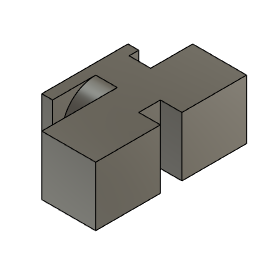
wire_screw v2 (Autodesk Fusion 360 design; units mm, degrees)
Autodesk Fusion 360 part; units mm, degrees
ref_plane "WorkPlane1" through (11.25, 0, 0) normal (1, 0, 0) x (0, 1, 0)
sketch "wire_screw2" plane through (0, 0, 0) normal (1, 0, 0) x (0, 1, 0)
  line L0 (7, 3.1) -> (-7, -3.1) construction
  line L1 (-7, 3.1) -> (7, -3.1) construction
  line L2 (-4, 4) -> (-4, -3.4897)
  line L3 (4, 4) -> (4, -3.5621)
  circle A0 centre (0, 0) radius 3.1
  circle A1 centre (0, 0) radius 2.75
  line L4 (-3.0288, -3.6864) -> (-3.0994, -0.0604)
  arc A2 (0, 2.75) -> (-3.0994, -0.0604) centre (0, -0.3643) ccw
  arc A3 (0, -2.75) -> (0, 2.75) centre (0, 0) ccw
  arc A4 (0, -2.75) -> (3.1, 0) centre (0, 0.3723) ccw
  line L5 (3.1, 0) -> (3.1, 3.8294)
  line L6 (0, 2.75) -> (3.1, 2.75)
  line L7 (0, -2.75) -> (-3.047, -2.75)
  line L8 (0, 2.75) -> (7, 2.75)
  line L9 (7, 2.75) -> (-7, 2.75)
  line L10 (-7, 2.75) -> (-7, -2.75)
  line L11 (-7, -2.75) -> (7, -2.75)
  line L12 (7, -2.75) -> (7, 2.75)
  dimension "d38" = 14
  dimension "d39" = 6.2
  dimension "d40" = 5.5
  dimension "d41" = 7
  dimension "d42" = 14
  constraint coincident A0.centre A1.centre
  constraint coincident L0 A0.centre
  constraint coincident L1 A0.centre
  constraint concentric A0 A1
  constraint coincident A0 L4.end
  constraint tangent A0 L4
  constraint tangent A1 A2
  constraint coincident A1 A2.start
  constraint tangent A1 A4
  constraint coincident A0 A4.end
  constraint tangent A0 L5
  constraint coincident L5 L6.end
  constraint tangent A1 L6
  constraint perpendicular L5 L6
  constraint coincident L4 L7.end
  constraint tangent A1 L7
  constraint horizontal L7
  constraint perpendicular L3 L8
  constraint horizontal L9
  constraint vertical L10
  constraint horizontal L11
  constraint vertical L12
  measures "d38" distance of L0.end L1.end
  measures "d39" diameter of A0
  measures "d40" diameter of A1
  measures "d41" distance of A2.start L8.end
  measures "d42" distance of L8.end L9.end
extrude "Extrude7" add sketch "wire_screw2" along normal blind -2 and the other way blind 3 contours L2 A0 L4 L9 L11 | A0 A2 L9 | A0 L4 L7 L11 | A0 L5 L6 L8 L9 | A0 A1 A3 A4 L6 L8 L9 | A0 A1 A2 L7 L11 | A1 A3 | L3 A0 L5 L8 L9 L11 | A0 A4 L11
extrude "Extrude8" add sketch "wire_screw2" against normal blind 2 contours A0 L4 L7 L11 | A0 L5 L6 L8 L9 | A0 A1 A3 A4 L6 L8 L9 | A0 A1 A2 L7 L11 | A1 A3
extrude "Extrude9" add sketch "wire_screw2" along normal blind 5 contours L2 A0 L4 L9 L11 | L2 L9 L10 L11 | A0 A2 L9 | A0 L4 L7 L11 | A0 L5 L6 L8 L9 | A0 A1 A3 A4 L6 L8 L9 | A0 A1 A2 L7 L11 | A1 A3 | L3 A0 L5 L8 L9 L11 | A0 A4 L11 | L3 L8 L9 L11 L12
sketch "wire_screw2_slot" plane through (0, 0, -2.75) normal (0, 0, -1) x (1, 0, 0)
  line L0 (-2, -4) -> (-2, 0)
  line L1 (-2, 0) -> (0, 0)
  line L2 (0, 0) -> (0, -7)
  line L3 (0, -7) -> (5, -7)
  line L4 (5, -7) -> (5, 7)
  line L5 (5, 7) -> (0, 7)
  line L6 (0, 7) -> (0, 3.047)
  line L7 (0, 3.047) -> (-2, 3.047)
  line L8 (-2, 3.047) -> (-2, 4)
  line L9 (-2, 4) -> (-3, 4)
  line L10 (-3, 4) -> (-3, -4)
  line L11 (-3, -4) -> (-2, -4)
  line L12 (3, 1) -> (7, 1)
  line L13 (7, 1) -> (7, -1)
  line L14 (7, -1) -> (3, -1)
  line L15 (3, -1) -> (3, 1)
  line L16 (3, 1) -> (7, -1) construction
  line L17 (7, 1) -> (3, -1) construction
  point P0 (5, 0)
  dimension "d51" = 4
  dimension "d52" = 2
  constraint horizontal L12
  constraint perpendicular L12 L13
  constraint parallel L12 L14
  constraint parallel L13 L15
  constraint coincident L16 P0
  constraint coincident L17 P0
  constraint midpoint L4 P0
  measures "d51" distance of L13.end L14.end
  measures "d52" distance of L12.end L13.end
extrude "Extrude10" cut sketch "wire_screw2_slot" against normal blind 8 contours L4 L12 L14 L15
named bodies: "wire_screw2"
